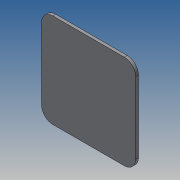
# Autodesk Inventor part: ground
Saved by Autodesk Inventor 2015 SP1 (Build 190203100, 203)
## iProperties
Created: 2015-12-28
Part Number: ground
Material: Generic
Document SubType Name: Modeling
Designer: Florian
Density: 1 g/cm^3
Appearance: Default
Author: Florian
Autodesk Inventor part; units mm, degrees
ref_plane "YZ Plane" through (0, 0, 0) normal (1, 0, 0) x (0, 1, 0)
ref_plane "XZ Plane" through (0, 0, 0) normal (0, 1, 0) x (-1, 0, 0)
ref_plane "XY Plane" through (0, 0, 0) normal (0, 0, 1) x (1, 0, 0)
sketch "Sketch1" plane through (0, 0, 0) normal (0, 1, 0) x (-1, 0, 0)
  line L0 (500, 500) -> (-500, 500)
  line L1 (-500, 500) -> (-500, -500)
  line L2 (-500, -500) -> (500, -500)
  line L3 (500, -500) -> (500, 500)
  point P0 (0, 0)
  point P1 (0, 500)
  point P2 (500, 0)
  dimension "d1" = 1000
  dimension "d2" = 1000
  constraints: 8 end point, 2 midpoint, 2 parallel, 1 horizontal, 1 horizontal alignment, 1 perpendicular, 1 vertical alignment
  measures "d1" distance of L0.start L0.end
  measures "d2" distance of L0.end L1.end
extrude "Extrusion1" add sketch "Sketch1" along normal blind 10
sketch "Sketch2" plane through (0, 10, 0) normal (0, 1, 0) x (1, 0, 0)
  line L0 (-480, -480) -> (480, -480)
  line L1 (480, -480) -> (480, 480)
  line L2 (480, 480) -> (-480, 480)
  line L3 (-480, 480) -> (-480, -480)
  line L4 (-500, 500) -> (-500, -500) projected
  line L5 (-500, -500) -> (500, -500) projected
  line L6 (500, -500) -> (500, 500) projected
  line L7 (500, 500) -> (-500, 500) projected
  point P0 (0, 0)
  dimension "d5" = 20
  dimension "d6" = 20
  dimension "d8" = 20
  dimension "d9" = 20
  constraints: 8 end point, 2 parallel, 1 horizontal, 1 perpendicular
  measures "d5" distance between parallel lines of L4 L3
  measures "d6" distance between parallel lines of L5 L0
  measures "d8" distance between parallel lines of L6 L1
  measures "d9" distance between parallel lines of L2 L7
extrude "Extrusion2" add sketch "Sketch2" along normal blind 20
fillet "Fillet1" radius 100 4 edges at (-480, 20, 480) (-480, 20, -480) (480, 20, -480) (480, 20, 480)
fillet "Fillet2" radius 120 4 edges at (-500, 15, 500) (-500, 15, -500) (500, 15, -500) (500, 15, 500)
equation "\"d6\" = d5"
equation "\"d8\" = d5"
equation "\"d9\" = d5"
body "Solid1"
